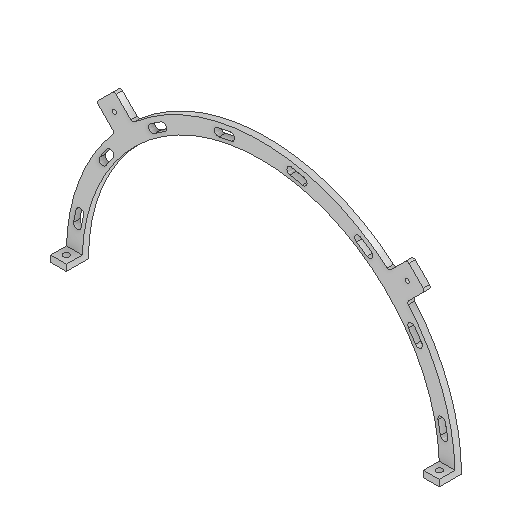
# Autodesk Inventor part: half_ring_1
Saved by Autodesk Inventor 2026.1 (Build 301233000, 233)
## iProperties
Created: 2025-09-17
Part Number: half_ring_1
Material: Aluminum 6061
Document SubType Name: Modeling
Designer: drago
Density: 2.7 g/cm^3
Appearance: Aluminum - Polished
Mass: 433.666 g
Surface Area: 584.563 cm^2
Volume: 160.617 cm^3
Author: drago
Autodesk Inventor part; units mm, degrees
ref_plane "YZ Plane" through (0, 0, 0) normal (1, 0, 0) x (0, 1, 0)
ref_plane "XZ Plane" through (0, 0, 0) normal (0, 1, 0) x (-1, 0, 0)
ref_plane "XY Plane" through (0, 0, 0) normal (0, 0, 1) x (1, 0, 0)
sketch "Sketch1" plane through (0, 0, 0) normal (0, 0, 1) x (1, 0, 0)
  circle A0 centre (0, 0) radius 307.5
  circle A1 centre (0, 0) radius 270.5 construction
  circle A2 centre (0, 0) radius 280.5 construction
  circle A3 centre (0, 0) radius 282.5
  line L0 (-307.5, 0) -> (307.5, 0)
  circle A4 centre (0, 0) radius 293.8 construction
  line L1 (0, 0) -> (307.3319, 10.1653) construction
  line L2 (0, 0) -> (-307.3319, 10.1653) construction
  line L3 (0, 0) -> (293.8, 0) construction
  line L4 (-307.3319, 10.1653) -> (307.3319, 10.1653)
  line L5 (0, 0) -> (301.5915, 59.9903) construction
  line L6 (0, 0) -> (307.5, 0) construction
  circle A5 centre (288.1547, 57.3175) radius 5 construction
  arc A6 (289.9795, 47.2262) -> (285.9788, 67.3391) centre (0, 0) ccw construction
  arc A7 (295.9015, 48.1906) -> (291.8191, 68.7143) centre (0, 0) ccw
  arc A8 (284.0576, 46.2617) -> (280.1386, 65.9639) centre (0, 0) ccw
  arc A9 (284.0576, 46.2617) -> (295.9015, 48.1906) centre (289.9795, 47.2262) ccw
  arc A10 (291.8191, 68.7143) -> (280.1386, 65.9639) centre (285.9788, 67.3391) ccw
  line L7 (0, 0) -> (289.9795, 47.2262) construction
  line L8 (0, 0) -> (293.8, 0) construction
  line L9 (0, 0) -> (285.9788, 67.3391) construction
  arc A11 (243.3099, 175.158) -> (233.571, 168.1471) centre (238.4404, 171.6526) ccw
  arc A12 (254.9356, 157.7589) -> (243.3099, 175.158) centre (0, 0) ccw
  arc A13 (244.7314, 151.4444) -> (233.571, 168.1471) centre (0, 0) ccw
  circle A14 centre (244.2858, 163.2265) radius 5 construction
  arc A15 (244.7314, 151.4444) -> (254.9356, 157.7589) centre (249.8335, 154.6017) ccw
  arc A16 (157.7589, 254.9356) -> (151.4444, 244.7314) centre (154.6017, 249.8335) ccw
  arc A17 (175.158, 243.3099) -> (157.7589, 254.9356) centre (0, 0) ccw
  arc A18 (168.1471, 233.571) -> (151.4444, 244.7314) centre (0, 0) ccw
  circle A19 centre (163.2265, 244.2858) radius 5 construction
  arc A20 (168.1471, 233.571) -> (175.158, 243.3099) centre (171.6526, 238.4404) ccw
  arc A21 (48.1906, 295.9015) -> (46.2617, 284.0576) centre (47.2262, 289.9795) ccw
  arc A22 (68.7143, 291.8191) -> (48.1906, 295.9015) centre (0, 0) ccw
  arc A23 (65.9639, 280.1386) -> (46.2617, 284.0576) centre (0, 0) ccw
  circle A24 centre (57.3175, 288.1547) radius 5 construction
  arc A25 (65.9639, 280.1386) -> (68.7143, 291.8191) centre (67.3391, 285.9788) ccw
  arc A26 (-68.7143, 291.8191) -> (-65.9639, 280.1386) centre (-67.3391, 285.9788) ccw
  arc A27 (-48.1906, 295.9015) -> (-68.7143, 291.8191) centre (0, 0) ccw
  arc A28 (-46.2617, 284.0576) -> (-65.9639, 280.1386) centre (0, 0) ccw
  circle A29 centre (-57.3175, 288.1547) radius 5 construction
  arc A30 (-46.2617, 284.0576) -> (-48.1906, 295.9015) centre (-47.2262, 289.9795) ccw
  arc A31 (-175.158, 243.3099) -> (-168.1471, 233.571) centre (-171.6526, 238.4404) ccw
  arc A32 (-157.7589, 254.9356) -> (-175.158, 243.3099) centre (0, 0) ccw
  arc A33 (-151.4444, 244.7314) -> (-168.1471, 233.571) centre (0, 0) ccw
  circle A34 centre (-163.2265, 244.2858) radius 5 construction
  arc A35 (-151.4444, 244.7314) -> (-157.7589, 254.9356) centre (-154.6017, 249.8335) ccw
  arc A36 (-254.9356, 157.7589) -> (-244.7314, 151.4444) centre (-249.8335, 154.6017) ccw
  arc A37 (-243.3099, 175.158) -> (-254.9356, 157.7589) centre (0, 0) ccw
  arc A38 (-233.571, 168.1471) -> (-244.7314, 151.4444) centre (0, 0) ccw
  circle A39 centre (-244.2858, 163.2265) radius 5 construction
  arc A40 (-233.571, 168.1471) -> (-243.3099, 175.158) centre (-238.4404, 171.6526) ccw
  arc A41 (-295.9015, 48.1906) -> (-284.0576, 46.2617) centre (-289.9795, 47.2262) ccw
  arc A42 (-291.8191, 68.7143) -> (-295.9015, 48.1906) centre (0, 0) ccw
  arc A43 (-280.1386, 65.9639) -> (-284.0576, 46.2617) centre (0, 0) ccw
  circle A44 centre (-288.1547, 57.3175) radius 5 construction
  arc A45 (-280.1386, 65.9639) -> (-291.8191, 68.7143) centre (-285.9788, 67.3391) ccw
  arc A46 (-291.8191, -68.7143) -> (-280.1386, -65.9639) centre (-285.9788, -67.3391) ccw
  arc A47 (-295.9015, -48.1906) -> (-291.8191, -68.7143) centre (0, 0) ccw
  arc A48 (-284.0576, -46.2617) -> (-280.1386, -65.9639) centre (0, 0) ccw
  circle A49 centre (-288.1547, -57.3175) radius 5 construction
  arc A50 (-284.0576, -46.2617) -> (-295.9015, -48.1906) centre (-289.9795, -47.2262) ccw
  arc A51 (-243.3099, -175.158) -> (-233.571, -168.1471) centre (-238.4404, -171.6526) ccw
  arc A52 (-254.9356, -157.7589) -> (-243.3099, -175.158) centre (0, 0) ccw
  arc A53 (-244.7314, -151.4444) -> (-233.571, -168.1471) centre (0, 0) ccw
  circle A54 centre (-244.2858, -163.2265) radius 5 construction
  arc A55 (-244.7314, -151.4444) -> (-254.9356, -157.7589) centre (-249.8335, -154.6017) ccw
  arc A56 (-157.7589, -254.9356) -> (-151.4444, -244.7314) centre (-154.6017, -249.8335) ccw
  arc A57 (-175.158, -243.3099) -> (-157.7589, -254.9356) centre (0, 0) ccw
  arc A58 (-168.1471, -233.571) -> (-151.4444, -244.7314) centre (0, 0) ccw
  circle A59 centre (-163.2265, -244.2858) radius 5 construction
  arc A60 (-168.1471, -233.571) -> (-175.158, -243.3099) centre (-171.6526, -238.4404) ccw
  arc A61 (-48.1906, -295.9015) -> (-46.2617, -284.0576) centre (-47.2262, -289.9795) ccw
  arc A62 (-68.7143, -291.8191) -> (-48.1906, -295.9015) centre (0, 0) ccw
  arc A63 (-65.9639, -280.1386) -> (-46.2617, -284.0576) centre (0, 0) ccw
  circle A64 centre (-57.3175, -288.1547) radius 5 construction
  arc A65 (-65.9639, -280.1386) -> (-68.7143, -291.8191) centre (-67.3391, -285.9788) ccw
  arc A66 (68.7143, -291.8191) -> (65.9639, -280.1386) centre (67.3391, -285.9788) ccw
  arc A67 (48.1906, -295.9015) -> (68.7143, -291.8191) centre (0, 0) ccw
  arc A68 (46.2617, -284.0576) -> (65.9639, -280.1386) centre (0, 0) ccw
  circle A69 centre (57.3175, -288.1547) radius 5 construction
  arc A70 (46.2617, -284.0576) -> (48.1906, -295.9015) centre (47.2262, -289.9795) ccw
  arc A71 (175.158, -243.3099) -> (168.1471, -233.571) centre (171.6526, -238.4404) ccw
  arc A72 (157.7589, -254.9356) -> (175.158, -243.3099) centre (0, 0) ccw
  arc A73 (151.4444, -244.7314) -> (168.1471, -233.571) centre (0, 0) ccw
  circle A74 centre (163.2265, -244.2858) radius 5 construction
  arc A75 (151.4444, -244.7314) -> (157.7589, -254.9356) centre (154.6017, -249.8335) ccw
  arc A76 (254.9356, -157.7589) -> (244.7314, -151.4444) centre (249.8335, -154.6017) ccw
  arc A77 (243.3099, -175.158) -> (254.9356, -157.7589) centre (0, 0) ccw
  arc A78 (233.571, -168.1471) -> (244.7314, -151.4444) centre (0, 0) ccw
  circle A79 centre (244.2858, -163.2265) radius 5 construction
  arc A80 (233.571, -168.1471) -> (243.3099, -175.158) centre (238.4404, -171.6526) ccw
  arc A81 (295.9015, -48.1906) -> (284.0576, -46.2617) centre (289.9795, -47.2262) ccw
  arc A82 (291.8191, -68.7143) -> (295.9015, -48.1906) centre (0, 0) ccw
  arc A83 (280.1386, -65.9639) -> (284.0576, -46.2617) centre (0, 0) ccw
  circle A84 centre (288.1547, -57.3175) radius 5 construction
  arc A85 (280.1386, -65.9639) -> (291.8191, -68.7143) centre (285.9788, -67.3391) ccw
  circle A86 centre (0, 0) radius 302.5 construction
  line L10 (347.5, -347.5) -> (-347.5, -347.5) construction
  line L11 (-347.5, -347.5) -> (-347.5, 347.5) construction
  line L12 (-347.5, 347.5) -> (347.5, 347.5) construction
  line L13 (347.5, 347.5) -> (347.5, -347.5) construction
  line L14 (347.5, -347.5) -> (-347.5, 347.5) construction
  line L15 (-347.5, -347.5) -> (347.5, 347.5) construction
  circle A87 centre (0, 0) radius 327.5 construction
  circle A88 centre (-231.5775, 231.5775) radius 3.4
  circle A89 centre (0, 0) radius 347.5 construction
  line L16 (-259.8617, 231.5775) -> (-231.5775, 259.8617)
  line L17 (-231.5775, 259.8617) -> (-202.8328, 231.1171)
  line L18 (-259.8617, 231.5775) -> (-231.1171, 202.8328)
  line L19 (-231.5775, -259.8617) -> (-259.8617, -231.5775)
  line L20 (-259.8617, -231.5775) -> (-231.1171, -202.8328)
  line L21 (-231.5775, -259.8617) -> (-202.8328, -231.1171)
  circle A90 centre (-231.5775, -231.5775) radius 3.4
  line L22 (259.8617, -231.5775) -> (231.5775, -259.8617)
  line L23 (231.5775, -259.8617) -> (202.8328, -231.1171)
  line L24 (259.8617, -231.5775) -> (231.1171, -202.8328)
  circle A91 centre (231.5775, -231.5775) radius 3.4
  line L25 (231.5775, 259.8617) -> (259.8617, 231.5775)
  line L26 (259.8617, 231.5775) -> (231.1171, 202.8328)
  line L27 (231.5775, 259.8617) -> (202.8328, 231.1171)
  circle A92 centre (231.5775, 231.5775) radius 3.4
  point P0 (282.5, 0)
  point P1 (307.5, 0)
  point P2 (-282.5, 0)
  point P3 (-282.3456, 9.3388)
  point P4 (282.3456, 9.3388)
  point P5 (282.3171, 10.1653)
  point P6 (-282.3171, 10.1653)
  point P7 (-245.7196, 245.7196)
  point P8 (231.1171, 202.8328)
  dimension "d70" = 695
  dimension "ring_outer_diam" = 615
  dimension "ring_inner_diam" = 565
  dimension "ring_cut_line" = 615
  dimension "help_line_length" = 307.5
  dimension "hole_angle_1" = 9.25
  dimension "hole_angle_2" = 4
  dimension "hole_diam" = 12
  dimension "d43" = 360
  dimension "d63" = 695
  dimension "d64" = 695
  dimension "d66" = 655
  dimension "d69" = 6.8
  dimension "d71" = 40
  dimension "d74" = 20
  dimension "d75" = 40
  dimension "d78" = 360
  constraints: 136 point on circle, 92 centre point, 56 end point, 10 coincident, 6 horizontal, 4 midpoint, 4 tangent, 3 equal length, 2 parallel, 2 perpendicular, 2 point on line, 255 other
  measures "ring_outer_diam" diameter of A0
  measures "ring_inner_diam" diameter of A3
  measures "ring_cut_line" distance of L0.start L0.end
  measures "help_line_length" distance of L3.start L5.end
  measures "hole_angle_1" angle of L8 L7
  measures "hole_angle_2" angle of L7 L9
  measures "hole_diam" diameter of A10
  measures "d63" distance of L11.end L12.end
  measures "d64" distance of L10.end L11.end
  measures "d66" diameter of A87
  measures "d69" diameter of A88
  measures "d71" distance of L16.start L16.end
  measures "d74" distance from line of L16 A88.centre
  measures "d75" distance between parallel lines of L18 L17
extrude "Extrusion1" add sketch "Sketch1" against normal blind 10 contours L0 A3 L4 A0 | L4 A3 A0 | L0 A0 L4 A3 | A9 A8 A10 A7 | A12 A15 A13 A11 | A17 A20 A18 A16 | A22 A25 A23 A21 | A27 A30 A28 A26 | A32 A35 A33 A31 | A37 A40 A38 A36 | A42 A45 A43 A41
extrude "Extrusion3" cut sketch "Sketch1" against normal blind 10 contours A9 A8 A10 A7 | A12 A15 A13 A11 | A17 A20 A18 A16 | A22 A25 A23 A21 | A27 A30 A28 A26 | A32 A35 A33 A31 | A37 A40 A38 A36 | A42 A45 A43 A41
extrude "Extrusion4" add sketch "Sketch1" along normal blind 25 contours L0 A3 L4 A0 | L0 A0 L4 A3
sketch "Sketch3" plane through (-307.5, 0, -10) normal (0, -1, 0) x (1, 0, 0)
  circle A0 centre (12.5, 22.5) radius 5
  line L0 (0, 35) -> (25, 35) projected
  line L1 (0, 0) -> (0, 35) projected
  circle A1 centre (602.5, 22.5) radius 5
  line L2 (590, 35) -> (615, 35) projected
  line L3 (615, 35) -> (615, 0) projected
  point P0 (307.5, 10)
  dimension "d49" = 10
  dimension "foot_hole_vert_pos" = 12.5
  dimension "foot_hole_horiz_pos" = 12.5
  dimension "d52" = 10
  dimension "d53" = 12.5
  dimension "d54" = 12.5
  constraints: 2 centre point
  measures "d49" diameter of A0
  measures "foot_hole_vert_pos" distance from line of A0.centre L0
  measures "foot_hole_horiz_pos" distance from line of L1 A0.centre
  measures "d52" diameter of A1
  measures "d53" distance from line of L2 A1.centre
  measures "d54" distance from line of L3 A1.centre
hole "Hole2" at (-295, 0, 12.5) at (295, 0, 12.5) direction (0, 1, 0) diameter 10 end through all
extrude "Extrusion5" add sketch "Sketch1" against normal blind 10 contours A0 L27 L25 L26 | A0 L18 L16 L17
fillet "Fillet1" radius 4 8 edges at (-231.5775, 259.8617, -5) (-202.8328, 231.1171, -5) (-259.8617, 231.5775, -5) (-231.1171, 202.8328, -5) (231.1171, 202.8328, -5) (259.8617, 231.5775, -5) (231.5775, 259.8617, -5) (202.8328, 231.1171, -5)
equation "\"ring_cut_line\" = ring_outer_diam"
equation "\"help_line_length\" = 0.5 * ring_outer_diam"
equation "\"foot_hole_vert_pos\" = 0.5 * foot_height"
equation "\"bar_screw_hole_diam\" = 6.8"
equation "\"foot_height\" = 25"
body "Solid1"
